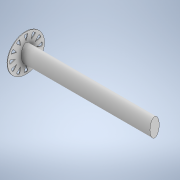
# Autodesk Inventor part: tanjiro's sword hold
Saved by Autodesk Inventor 2022 (Build 260153000, 153)
## iProperties
Created: 2022-01-01
Part Number: tanjiro's sword hold
Material: Generic
Document SubType Name: Modeling
Designer: saipr
Density: 1 g/cm^3
Appearance: Default
Author: saipr
Autodesk Inventor part; units mm, degrees
ref_plane "YZ Plane" through (0, 0, 0) normal (1, 0, 0) x (0, 1, 0)
ref_plane "XZ Plane" through (0, 0, 0) normal (0, 1, 0) x (-1, 0, 0)
ref_plane "XY Plane" through (0, 0, 0) normal (0, 0, 1) x (1, 0, 0)
sketch "Sketch4" plane through (0, 0, 0) normal (1, 0, 0) x (0, 1, 0)
  ellipse E0 centre (0, 0) end of major axis (-20, 0) minor radius 10
  dimension "d32" = 20
  dimension "d33" = 10
  constraints: 1 coincident, 2 other
extrude "Extrusion1" add sketch "Sketch4" along normal blind 280
sketch "Sketch5" plane through (0, 0, 0) normal (-1, 0, 0) x (0, 0, 1)
  ellipse E0 centre (0, 0) end of major axis (0, 40) minor radius 40
  ellipse E1 centre (0, 0) end of major axis (0, -20) minor radius 10 projected
  line L0 (0, 0) -> (0, 40)
  line L1 (0, 0) -> (-20, 34.641)
  line L2 (0, 0) -> (-34.641, 20)
  line L3 (0, 0) -> (-40, 0)
  line L4 (0, 0) -> (-34.641, -20)
  line L5 (0, 0) -> (-20, -34.641)
  line L6 (0, 0) -> (0, -40)
  line L7 (0, 0) -> (20, -34.641)
  line L8 (0, 0) -> (34.641, -20)
  line L9 (0, 0) -> (40, 0)
  line L10 (0, 0) -> (34.641, 20)
  line L11 (0, 0) -> (20, 34.641)
  line L12 (0, 23.094) -> (3.6979, 33.254)
  line L13 (2.2062, 35.3845) -> (0, 35.3845)
  arc A0 (3.6979, 33.254) -> (2.2062, 35.3845) centre (2.2062, 33.797) ccw
  line L14 (0, 23.094) -> (-3.6979, 33.254)
  line L15 (-2.2062, 35.3845) -> (0, 35.3845)
  arc A1 (-2.2062, 35.3845) -> (-3.6979, 33.254) centre (-2.2062, 33.797) ccw
  line L16 (-15.7816, 31.7469) -> (-17.6922, 30.6438)
  line L17 (-19.6028, 29.5408) -> (-17.6922, 30.6438)
  arc A2 (-19.6028, 29.5408) -> (-19.8295, 26.9498) centre (-18.8091, 28.1659) ccw
  line L18 (-11.547, 20) -> (-19.8295, 26.9498)
  line L19 (-11.547, 20) -> (-13.4245, 30.6478)
  arc A3 (-13.4245, 30.6478) -> (-15.7816, 31.7469) centre (-14.9879, 30.3721) ccw
  line L20 (-29.5408, 19.6028) -> (-30.6438, 17.6922)
  line L21 (-31.7469, 15.7816) -> (-30.6438, 17.6922)
  arc A4 (-31.7469, 15.7816) -> (-30.6478, 13.4245) centre (-30.3721, 14.9879) ccw
  line L22 (-20, 11.547) -> (-30.6478, 13.4245)
  line L23 (-20, 11.547) -> (-26.9498, 19.8295)
  arc A5 (-26.9498, 19.8295) -> (-29.5408, 19.6028) centre (-28.1659, 18.8091) ccw
  line L24 (-35.3845, 2.2062) -> (-35.3845, 0)
  line L25 (-35.3845, -2.2062) -> (-35.3845, 0)
  arc A6 (-35.3845, -2.2062) -> (-33.254, -3.6979) centre (-33.797, -2.2062) ccw
  line L26 (-23.094, 0) -> (-33.254, -3.6979)
  line L27 (-23.094, 0) -> (-33.254, 3.6979)
  arc A7 (-33.254, 3.6979) -> (-35.3845, 2.2062) centre (-33.797, 2.2062) ccw
  line L28 (-31.7469, -15.7816) -> (-30.6438, -17.6922)
  line L29 (-29.5408, -19.6028) -> (-30.6438, -17.6922)
  arc A8 (-29.5408, -19.6028) -> (-26.9498, -19.8295) centre (-28.1659, -18.8091) ccw
  line L30 (-20, -11.547) -> (-26.9498, -19.8295)
  line L31 (-20, -11.547) -> (-30.6478, -13.4245)
  arc A9 (-30.6478, -13.4245) -> (-31.7469, -15.7816) centre (-30.3721, -14.9879) ccw
  line L32 (-19.6028, -29.5408) -> (-17.6922, -30.6438)
  line L33 (-15.7816, -31.7469) -> (-17.6922, -30.6438)
  arc A10 (-15.7816, -31.7469) -> (-13.4245, -30.6478) centre (-14.9879, -30.3721) ccw
  line L34 (-11.547, -20) -> (-13.4245, -30.6478)
  line L35 (-11.547, -20) -> (-19.8295, -26.9498)
  arc A11 (-19.8295, -26.9498) -> (-19.6028, -29.5408) centre (-18.8091, -28.1659) ccw
  line L36 (-2.2062, -35.3845) -> (0, -35.3845)
  line L37 (2.2062, -35.3845) -> (0, -35.3845)
  arc A12 (2.2062, -35.3845) -> (3.6979, -33.254) centre (2.2062, -33.797) ccw
  line L38 (0, -23.094) -> (3.6979, -33.254)
  line L39 (0, -23.094) -> (-3.6979, -33.254)
  arc A13 (-3.6979, -33.254) -> (-2.2062, -35.3845) centre (-2.2062, -33.797) ccw
  line L40 (15.7816, -31.7469) -> (17.6922, -30.6438)
  line L41 (19.6028, -29.5408) -> (17.6922, -30.6438)
  arc A14 (19.6028, -29.5408) -> (19.8295, -26.9498) centre (18.8091, -28.1659) ccw
  line L42 (11.547, -20) -> (19.8295, -26.9498)
  line L43 (11.547, -20) -> (13.4245, -30.6478)
  arc A15 (13.4245, -30.6478) -> (15.7816, -31.7469) centre (14.9879, -30.3721) ccw
  line L44 (29.5408, -19.6028) -> (30.6438, -17.6922)
  line L45 (31.7469, -15.7816) -> (30.6438, -17.6922)
  arc A16 (31.7469, -15.7816) -> (30.6478, -13.4245) centre (30.3721, -14.9879) ccw
  line L46 (20, -11.547) -> (30.6478, -13.4245)
  line L47 (20, -11.547) -> (26.9498, -19.8295)
  arc A17 (26.9498, -19.8295) -> (29.5408, -19.6028) centre (28.1659, -18.8091) ccw
  line L48 (35.3845, -2.2062) -> (35.3845, 0)
  line L49 (35.3845, 2.2062) -> (35.3845, 0)
  arc A18 (35.3845, 2.2062) -> (33.254, 3.6979) centre (33.797, 2.2062) ccw
  line L50 (23.094, 0) -> (33.254, 3.6979)
  line L51 (23.094, 0) -> (33.254, -3.6979)
  arc A19 (33.254, -3.6979) -> (35.3845, -2.2062) centre (33.797, -2.2062) ccw
  line L52 (31.7469, 15.7816) -> (30.6438, 17.6922)
  line L53 (29.5408, 19.6028) -> (30.6438, 17.6922)
  arc A20 (29.5408, 19.6028) -> (26.9498, 19.8295) centre (28.1659, 18.8091) ccw
  line L54 (20, 11.547) -> (26.9498, 19.8295)
  line L55 (20, 11.547) -> (30.6478, 13.4245)
  arc A21 (30.6478, 13.4245) -> (31.7469, 15.7816) centre (30.3721, 14.9879) ccw
  line L56 (19.6028, 29.5408) -> (17.6922, 30.6438)
  line L57 (15.7816, 31.7469) -> (17.6922, 30.6438)
  arc A22 (15.7816, 31.7469) -> (13.4245, 30.6478) centre (14.9879, 30.3721) ccw
  line L58 (11.547, 20) -> (13.4245, 30.6478)
  line L59 (11.547, 20) -> (19.8295, 26.9498)
  arc A23 (19.8295, 26.9498) -> (19.6028, 29.5408) centre (18.8091, 28.1659) ccw
  line L60 (-3.175, 3.5066) -> (3.175, 3.5066)
  line L61 (3.175, 3.5066) -> (3.175, -3.5066)
  line L62 (3.175, -3.5066) -> (-3.175, -3.5066)
  line L63 (-3.175, -3.5066) -> (-3.175, 3.5066)
  line L64 (-3.175, 3.5066) -> (3.175, -3.5066) construction
  line L65 (3.175, 3.5066) -> (-3.175, -3.5066) construction
  dimension "d36" = 40
  dimension "d40" = 40
  dimension "d43" = 360
  dimension "d45" = 1.5875
  dimension "d46" = 10.16
  dimension "d47" = 20
  dimension "d50" = 360
  dimension "d52" = 6.35
  constraints: 132 end point, 48 point on circle, 24 centre point, 3 coincident, 3 symmetric about line, 2 midpoint, 2 parallel, 2 perpendicular, 2 point on line, 2 tangent, 1 horizontal, 1 vertical, 1 vertical alignment, 220 other
  measures "d45" radius of A0
  measures "d46" vertical distance of L12.start L12.end
  measures "d47" angle of L0 L12
  measures "d52" distance of L60.start L60.end
extrude "Extrusion2" add sketch "Sketch5" against normal blind 1.25 contours L0 L15 A1 L14 E1 L1 L19 A3 L16 E0 | E0 L11 L57 A22 L58 E1 L0 L12 A0 L13 | L1 L17 A2 L18 E1 L2 L23 A5 L20 E0 | E0 L10 L53 A20 L54 E1 L11 L59 A23 L56 | L2 L21 A4 L22 E1 L3 L27 A7 L24 E0 | E0 L9 L49 A18 L50 E1 L10 L55 A21 L52 | L3 L25 A6 L26 E1 L4 L31 A9 L28 E0 | E0 L8 L45 A16 L46 E1 L9 L51 A19 L48 | L4 L29 A8 L30 E1 L5 L35 A11 L32 E0 | E0 L7 L41 A14 L42 E1 L8 L47 A17 L44 | L5 L33 A10 L34 E1 L6 L39 A13 L36 E0 | E0 L6 L37 A12 L38 E1 L7 L43 A15 L40
extrude "Extrusion3" cut sketch "Sketch5" against normal blind 6.35 contours L60 L11 L0 | L0 L1 L60 | L1 L2 L63 L60 | L60 L61 L10 L11 | L3 L63 L2 | L4 L63 L3 | L5 L62 L63 L4 | L6 L62 L5 | L7 L62 L6 | L8 L61 L62 L7 | L9 L61 L8 | L10 L61 L9
equation "\"d33\" = 0.5 * d32"
equation "\"d36\" = d40"
body "Solid1"
